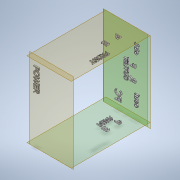
# Autodesk Inventor part: BaseTextWhite
Saved by Autodesk Inventor 2022 (Build 260153000, 153)
## iProperties
Created: 2022-01-15
Part Number: BaseTextWhite
Material: Generic
Document SubType Name: Modeling
Designer: siwat
Density: 1 g/cm^3
Appearance: Default
VLDS_Profile: Default Part
VLDS_TimeStamp: 2022-02-28
VLDS_FailCnt: 0
VLDS_AcceptCnt: 0
Author: siwat
Autodesk Inventor part; units mm, degrees
(part 1 of 2)
ref_plane "YZ Plane" through (0, 0, 0) normal (1, 0, 0) x (0, 1, 0)
ref_plane "XZ Plane" through (0, 0, 0) normal (0, 1, 0) x (-1, 0, 0)
ref_plane "XY Plane" through (0, 0, 0) normal (0, 0, 1) x (1, 0, 0)
ref_plane "Work Plane1" through (0, 0, 0) normal (0, 0, 1) x (1, 0, 0)
sketch "Sketch1" plane through (0, 0, 0) normal (0, 0, 1) x (1, 0, 0)
  line L0 (10.9128, -13.6781) -> (10.9128, -59.6425) construction
  line L1 (10.9128, -59.6425) -> (0.4914, -59.6425) construction
  line L2 (0.4914, -59.6425) -> (0.4914, -13.6781) construction
  line L3 (0.4914, -13.6781) -> (10.9128, -13.6781) construction
  spline S0 degree 2 poles (7.6875, -21.012) (7.0392, -21.012) (5.8723, -20.5501) (5.4671, -20.1368) knots 0 0 0 1 2 2 2
  spline S1 degree 2 poles (5.4671, -20.1368) (4.9565, -19.6182) (4.4298, -18.2162) (4.4298, -17.1465) knots 0 0 0 1 2 2 2
  line L4 (4.4298, -17.1465) -> (4.4298, -16.0201)
  line L5 (4.4298, -16.0201) -> (0.7021, -16.0201)
  line L6 (0.7021, -16.0201) -> (0.7021, -14.6911)
  line L7 (0.7021, -14.6911) -> (10.7021, -14.6911)
  line L8 (10.7021, -14.6911) -> (10.7021, -17.2032)
  spline S2 degree 2 poles (10.7021, -17.2032) (10.7021, -18.0947) (10.4104, -19.3426) (10.0781, -19.8207) knots 0 0 0 1 2 2 2
  spline S3 degree 2 poles (10.0781, -19.8207) (9.6972, -20.3799) (8.5222, -21.012) (7.6875, -21.012) knots 0 0 0 1 2 2 2
  spline S4 degree 2 poles (7.647, -19.6263) (8.1656, -19.6263) (8.9274, -19.2697) (9.1705, -18.905) knots 0 0 0 1 2 2 2
  spline S5 degree 2 poles (9.1705, -18.905) (9.3812, -18.589) (9.5514, -17.7462) (9.5514, -17.1222) knots 0 0 0 1 2 2 2
  line L9 (9.5514, -17.1222) -> (9.5514, -16.0201)
  line L10 (9.5514, -16.0201) -> (5.5643, -16.0201)
  line L11 (5.5643, -16.0201) -> (5.5643, -16.9277)
  spline S6 degree 2 poles (5.5643, -16.9277) (5.5643, -17.7381) (5.8236, -18.7348) (6.164, -19.059) knots 0 0 0 1 2 2 2
  spline S7 degree 2 poles (6.164, -19.059) (6.4638, -19.3588) (7.1689, -19.6263) (7.647, -19.6263) knots 0 0 0 1 2 2 2
  spline S8 degree 2 poles (9.5595, -29.3507) (8.895, -29.918) (6.9501, -30.5501) (5.7021, -30.5501) knots 0 0 0 1 2 2 2
  spline S9 degree 2 poles (5.7021, -30.5501) (4.4865, -30.5501) (2.5173, -29.9342) (1.8528, -29.3507) knots 0 0 0 1 2 2 2
  spline S10 degree 2 poles (1.8528, -29.3507) (1.1559, -28.7348) (0.4914, -27.106) (0.4914, -26.1254) knots 0 0 0 1 2 2 2
  spline S11 degree 2 poles (0.4914, -26.1254) (0.4914, -25.1125) (1.1802, -23.4917) (1.8528, -22.9002) knots 0 0 0 1 2 2 2
  spline S12 degree 2 poles (1.8528, -22.9002) (2.5173, -22.3248) (4.4703, -21.7089) (5.7021, -21.7089) knots 0 0 0 1 2 2 2
  spline S13 degree 2 poles (5.7021, -21.7089) (6.9582, -21.7089) (8.8706, -22.3329) (9.5595, -22.9083) knots 0 0 0 1 2 2 2
  spline S14 degree 2 poles (9.5595, -22.9083) (10.224, -23.4917) (10.9128, -25.1206) (10.9128, -26.1254) knots 0 0 0 1 2 2 2
  spline S15 degree 2 poles (10.9128, -26.1254) (10.9128, -27.1465) (10.1997, -28.7835) (9.5595, -29.3507) knots 0 0 0 1 2 2 2
  spline S16 degree 2 poles (5.7021, -29.1643) (6.6907, -29.1643) (8.2223, -28.7348) (8.7248, -28.3459) knots 0 0 0 1 2 2 2
  spline S17 degree 2 poles (8.7248, -28.3459) (9.2434, -27.9488) (9.7621, -26.8305) (9.7621, -26.1335) knots 0 0 0 1 2 2 2
  spline S18 degree 2 poles (9.7621, -26.1335) (9.7621, -25.4123) (9.2596, -24.3264) (8.7248, -23.9131) knots 0 0 0 1 2 2 2
  spline S19 degree 2 poles (8.7248, -23.9131) (8.2142, -23.516) (6.6745, -23.0947) (5.7021, -23.0947) knots 0 0 0 1 2 2 2
  spline S20 degree 2 poles (5.7021, -23.0947) (3.7329, -23.0947) (1.6421, -24.7478) (1.6421, -26.1335) knots 0 0 0 1 2 2 2
  spline S21 degree 2 poles (1.6421, -26.1335) (1.6421, -27.5193) (3.7329, -29.1643) (5.7021, -29.1643) knots 0 0 0 1 2 2 2
  line L12 (10.7021, -43.2162) -> (0.7021, -40.7041)
  line L13 (0.7021, -40.7041) -> (0.7021, -39.213)
  line L14 (0.7021, -39.213) -> (9.0003, -37.1789)
  line L15 (9.0003, -37.1789) -> (0.7021, -35.2016)
  line L16 (0.7021, -35.2016) -> (0.7021, -33.7267)
  line L17 (0.7021, -33.7267) -> (10.7021, -31.1741)
  line L18 (10.7021, -31.1741) -> (10.7021, -32.5436)
  line L19 (10.7021, -32.5436) -> (2.412, -34.5533)
  line L20 (2.412, -34.5533) -> (10.7021, -36.5468)
  line L21 (10.7021, -36.5468) -> (10.7021, -37.9002)
  line L22 (10.7021, -37.9002) -> (2.3147, -39.9099)
  line L23 (2.3147, -39.9099) -> (10.7021, -41.9115)
  line L24 (10.7021, -41.9115) -> (10.7021, -43.2162)
  line L25 (0.7021, -44.4075) -> (10.7021, -44.4075)
  line L26 (10.7021, -44.4075) -> (10.7021, -50.6635)
  line L27 (10.7021, -50.6635) -> (9.5189, -50.6635)
  line L28 (9.5189, -50.6635) -> (9.5189, -45.7365)
  line L29 (9.5189, -45.7365) -> (6.7799, -45.7365)
  line L30 (6.7799, -45.7365) -> (6.7799, -50.3313)
  line L31 (6.7799, -50.3313) -> (5.5967, -50.3313)
  line L32 (5.5967, -50.3313) -> (5.5967, -45.7365)
  line L33 (5.5967, -45.7365) -> (1.8852, -45.7365)
  line L34 (1.8852, -45.7365) -> (1.8852, -50.6635)
  line L35 (1.8852, -50.6635) -> (0.7021, -50.6635)
  line L36 (0.7021, -50.6635) -> (0.7021, -44.4075)
  line L37 (0.7021, -59.8613) -> (0.7021, -58.1352)
  line L38 (0.7021, -58.1352) -> (4.681, -54.9747)
  line L39 (4.681, -54.9747) -> (4.681, -53.4512)
  line L40 (4.681, -53.4512) -> (0.7021, -53.4512)
  line L41 (0.7021, -53.4512) -> (0.7021, -52.1222)
  line L42 (0.7021, -52.1222) -> (10.7021, -52.1222)
  line L43 (10.7021, -52.1222) -> (10.7021, -54.6992)
  spline S22 degree 2 poles (10.7021, -54.6992) (10.7021, -55.5582) (10.5157, -56.717) (10.1753, -57.2438) knots 0 0 0 1 2 2 2
  spline S23 degree 2 poles (10.1753, -57.2438) (9.835, -57.7705) (8.7734, -58.3783) (7.9873, -58.3783) knots 0 0 0 1 2 2 2
  spline S24 degree 2 poles (7.9873, -58.3783) (6.8933, -58.3783) (5.4104, -57.26) (5.0538, -56.3037) knots 0 0 0 1 2 2 2
  line L44 (5.0538, -56.3037) -> (0.7021, -59.8613)
  spline S25 degree 2 poles (7.882, -56.9925) (8.3196, -56.9925) (8.9922, -56.6846) (9.211, -56.3605) knots 0 0 0 1 2 2 2
  spline S26 degree 2 poles (9.211, -56.3605) (9.3974, -56.0768) (9.5514, -55.3232) (9.5514, -54.7721) knots 0 0 0 1 2 2 2
  line L45 (9.5514, -54.7721) -> (9.5514, -53.4512)
  line L46 (9.5514, -53.4512) -> (5.7912, -53.4512)
  line L47 (5.7912, -53.4512) -> (5.7912, -54.6182)
  spline S27 degree 2 poles (5.7912, -54.6182) (5.7912, -55.1935) (5.9938, -56.1092) (6.3099, -56.4253) knots 0 0 0 1 2 2 2
  spline S28 degree 2 poles (6.3099, -56.4253) (6.5854, -56.717) (7.3634, -56.9925) (7.882, -56.9925) knots 0 0 0 1 2 2 2
  point P0 (0, 0)
  constraints: 2 other
extrude "Extrusion1" add sketch "Sketch1" against normal blind 2
ref_plane "Work Plane2" through (-0.0003, -144.9621, -142.4319) normal (0, 0, -1) x (-1, 0, 0)
sketch "Sketch2" plane through (-0.0003, -144.9621, -142.4319) normal (0, 0, -1) x (-1, 0, 0)
  line L0 (-56.0033, 81.336) -> (-56.0033, 88.5078) construction
  line L1 (-56.0033, 88.5078) -> (-46.0033, 88.5078) construction
  line L2 (-46.0033, 88.5078) -> (-46.0033, 81.336) construction
  line L3 (-46.0033, 81.336) -> (-56.0033, 81.336) construction
  line L4 (-56.1337, 56.3409) -> (-56.1337, 65.1713) construction
  line L5 (-56.1337, 65.1713) -> (-45.8315, 65.1713) construction
  line L6 (-45.8315, 65.1713) -> (-45.8315, 56.3409) construction
  line L7 (-45.8315, 56.3409) -> (-56.1337, 56.3409) construction
  line L8 (-42.4083, 53.9471) -> (-42.4083, 111.4785) construction
  line L9 (-42.4083, 111.4785) -> (-33.0274, 111.4785) construction
  line L10 (-33.0274, 111.4785) -> (-33.0274, 53.9471) construction
  line L11 (-33.0274, 53.9471) -> (-42.4083, 53.9471) construction
  line L12 (-29.0759, 10.8608) -> (-29.0759, 68.3922) construction
  line L13 (-29.0759, 68.3922) -> (-19.695, 68.3922) construction
  line L14 (-19.695, 68.3922) -> (-19.695, 10.8608) construction
  line L15 (-19.695, 10.8608) -> (-29.0759, 10.8608) construction
  line L16 (-46.1337, 65.0929) -> (-46.1337, 63.3668)
  line L17 (-46.1337, 63.3668) -> (-50.1126, 60.2064)
  line L18 (-50.1126, 60.2064) -> (-50.1126, 58.6829)
  line L19 (-50.1126, 58.6829) -> (-46.1337, 58.6829)
  line L20 (-46.1337, 58.6829) -> (-46.1337, 57.3539)
  line L21 (-46.1337, 57.3539) -> (-56.1337, 57.3539)
  line L22 (-56.1337, 57.3539) -> (-56.1337, 59.9308)
  spline S0 degree 2 poles (-56.1337, 59.9308) (-56.1337, 60.7898) (-55.9473, 61.9487) (-55.6069, 62.4754) knots 0 0 0 1 2 2 2
  spline S1 degree 2 poles (-55.6069, 62.4754) (-55.2666, 63.0022) (-54.205, 63.6099) (-53.4189, 63.6099) knots 0 0 0 1 2 2 2
  spline S2 degree 2 poles (-53.4189, 63.6099) (-52.3249, 63.6099) (-50.8419, 62.4916) (-50.4854, 61.5354) knots 0 0 0 1 2 2 2
  line L23 (-50.4854, 61.5354) -> (-46.1337, 65.0929)
  spline S3 degree 2 poles (-53.3136, 62.2242) (-53.7512, 62.2242) (-54.4238, 61.9163) (-54.6426, 61.5921) knots 0 0 0 1 2 2 2
  spline S4 degree 2 poles (-54.6426, 61.5921) (-54.829, 61.3085) (-54.9829, 60.5548) (-54.9829, 60.0038) knots 0 0 0 1 2 2 2
  line L24 (-54.9829, 60.0038) -> (-54.9829, 58.6829)
  line L25 (-54.9829, 58.6829) -> (-51.2228, 58.6829)
  line L26 (-51.2228, 58.6829) -> (-51.2228, 59.8498)
  spline S5 degree 2 poles (-51.2228, 59.8498) (-51.2228, 60.4252) (-51.4254, 61.3409) (-51.7414, 61.6569) knots 0 0 0 1 2 2 2
  spline S6 degree 2 poles (-51.7414, 61.6569) (-52.017, 61.9487) (-52.7949, 62.2242) (-53.3136, 62.2242) knots 0 0 0 1 2 2 2
  line L27 (-54.8201, 88.3295) -> (-54.8201, 83.678)
  line L28 (-54.8201, 83.678) -> (-52, 83.678)
  line L29 (-52, 83.678) -> (-52, 88.135)
  line L30 (-52, 88.135) -> (-50.8169, 88.135)
  line L31 (-50.8169, 88.135) -> (-50.8169, 83.678)
  line L32 (-50.8169, 83.678) -> (-46.0033, 83.678)
  line L33 (-46.0033, 83.678) -> (-46.0033, 82.349)
  line L34 (-46.0033, 82.349) -> (-56.0033, 82.349)
  line L35 (-56.0033, 82.349) -> (-56.0033, 88.3295)
  line L36 (-56.0033, 88.3295) -> (-54.8201, 88.3295)
  spline S7 degree 2 poles (-41.3257, 60.4171) (-40.7941, 60.8709) (-39.2382, 61.3766) (-38.2398, 61.3766) knots 0 0 0 1 2 2 2
  spline S8 degree 2 poles (-38.2398, 61.3766) (-37.2673, 61.3766) (-35.692, 60.8839) (-35.1604, 60.4171) knots 0 0 0 1 2 2 2
  spline S9 degree 2 poles (-35.1604, 60.4171) (-34.6028, 59.9244) (-34.0712, 58.6213) (-34.0712, 57.8369) knots 0 0 0 1 2 2 2
  spline S10 degree 2 poles (-34.0712, 57.8369) (-34.0712, 57.0265) (-34.6223, 55.7299) (-35.1604, 55.2567) knots 0 0 0 1 2 2 2
  spline S11 degree 2 poles (-35.1604, 55.2567) (-35.692, 54.7964) (-37.2544, 54.3037) (-38.2398, 54.3037) knots 0 0 0 1 2 2 2
  spline S12 degree 2 poles (-38.2398, 54.3037) (-39.2446, 54.3037) (-40.7746, 54.8028) (-41.3257, 55.2631) knots 0 0 0 1 2 2 2
  spline S13 degree 2 poles (-41.3257, 55.2631) (-41.8573, 55.7299) (-42.4083, 57.033) (-42.4083, 57.8369) knots 0 0 0 1 2 2 2
  spline S14 degree 2 poles (-42.4083, 57.8369) (-42.4083, 58.6537) (-41.8378, 59.9633) (-41.3257, 60.4171) knots 0 0 0 1 2 2 2
  spline S15 degree 2 poles (-38.2398, 60.268) (-39.0307, 60.268) (-40.256, 59.9244) (-40.6579, 59.6132) knots 0 0 0 1 2 2 2
  spline S16 degree 2 poles (-40.6579, 59.6132) (-41.0728, 59.2956) (-41.4878, 58.4009) (-41.4878, 57.8434) knots 0 0 0 1 2 2 2
  spline S17 degree 2 poles (-41.4878, 57.8434) (-41.4878, 57.2664) (-41.0858, 56.3977) (-40.6579, 56.067) knots 0 0 0 1 2 2 2
  spline S18 degree 2 poles (-40.6579, 56.067) (-40.2495, 55.7494) (-39.0177, 55.4122) (-38.2398, 55.4122) knots 0 0 0 1 2 2 2
  spline S19 degree 2 poles (-38.2398, 55.4122) (-36.6644, 55.4122) (-34.9918, 56.7348) (-34.9918, 57.8434) knots 0 0 0 1 2 2 2
  spline S20 degree 2 poles (-34.9918, 57.8434) (-34.9918, 58.952) (-36.6644, 60.268) (-38.2398, 60.268) knots 0 0 0 1 2 2 2
  spline S21 degree 2 poles (-34.0712, 65.3377) (-34.0712, 64.631) (-34.4408, 63.5808) (-34.8103, 63.2113) knots 0 0 0 1 2 2 2
  spline S22 degree 2 poles (-34.8103, 63.2113) (-35.2252, 62.7899) (-36.3921, 62.4463) (-37.2479, 62.4463) knots 0 0 0 1 2 2 2
  line L37 (-37.2479, 62.4463) -> (-42.2398, 62.4463)
  line L38 (-42.2398, 62.4463) -> (-42.2398, 63.5095)
  line L39 (-42.2398, 63.5095) -> (-37.2479, 63.5095)
  spline S23 degree 2 poles (-37.2479, 63.5095) (-36.6904, 63.5095) (-35.9383, 63.6521) (-35.6336, 63.8531) knots 0 0 0 1 2 2 2
  spline S24 degree 2 poles (-35.6336, 63.8531) (-35.3095, 64.067) (-34.9788, 64.8061) (-34.9788, 65.3377) knots 0 0 0 1 2 2 2
  spline S25 degree 2 poles (-34.9788, 65.3377) (-34.9788, 65.8369) (-35.3095, 66.6148) (-35.6336, 66.8288) knots 0 0 0 1 2 2 2
  spline S26 degree 2 poles (-35.6336, 66.8288) (-35.9383, 67.0298) (-36.6839, 67.1724) (-37.222, 67.1724) knots 0 0 0 1 2 2 2
  line L40 (-37.222, 67.1724) -> (-42.2398, 67.1724)
  line L41 (-42.2398, 67.1724) -> (-42.2398, 68.2356)
  line L42 (-42.2398, 68.2356) -> (-37.2479, 68.2356)
  spline S27 degree 2 poles (-37.2479, 68.2356) (-36.4116, 68.2356) (-35.2187, 67.8985) (-34.8103, 67.4706) knots 0 0 0 1 2 2 2
  spline S28 degree 2 poles (-34.8103, 67.4706) (-34.4343, 67.0881) (-34.0712, 66.0768) (-34.0712, 65.3377) knots 0 0 0 1 2 2 2
  line L43 (-34.2398, 71.6262) -> (-41.2933, 71.6262)
  line L44 (-41.2933, 71.6262) -> (-41.2933, 68.9422)
  line L45 (-41.2933, 68.9422) -> (-42.2398, 68.9422)
  line L46 (-42.2398, 68.9422) -> (-42.2398, 75.3733)
  line L47 (-42.2398, 75.3733) -> (-41.2933, 75.3733)
  line L48 (-41.2933, 75.3733) -> (-41.2933, 72.6894)
  line L49 (-41.2933, 72.6894) -> (-34.2398, 72.6894)
  line L50 (-34.2398, 72.6894) -> (-34.2398, 71.6262)
  line L51 (-34.2398, 80.8191) -> (-34.2398, 76.1837)
  line L52 (-34.2398, 76.1837) -> (-42.2398, 76.1837)
  line L53 (-42.2398, 76.1837) -> (-42.2398, 77.2469)
  line L54 (-42.2398, 77.2469) -> (-35.1863, 77.2469)
  line L55 (-35.1863, 77.2469) -> (-35.1863, 80.8191)
  line L56 (-35.1863, 80.8191) -> (-34.2398, 80.8191)
  line L57 (-34.2398, 81.6554) -> (-42.2398, 81.6554)
  line L58 (-42.2398, 81.6554) -> (-42.2398, 86.6602)
  line L59 (-42.2398, 86.6602) -> (-41.2933, 86.6602)
  line L60 (-41.2933, 86.6602) -> (-41.2933, 82.7186)
  line L61 (-41.2933, 82.7186) -> (-39.102, 82.7186)
  line L62 (-39.102, 82.7186) -> (-39.102, 86.3944)
  line L63 (-39.102, 86.3944) -> (-38.1555, 86.3944)
  line L64 (-38.1555, 86.3944) -> (-38.1555, 82.7186)
  line L65 (-38.1555, 82.7186) -> (-35.1863, 82.7186)
  line L66 (-35.1863, 82.7186) -> (-35.1863, 86.6602)
  line L67 (-35.1863, 86.6602) -> (-34.2398, 86.6602)
  line L68 (-34.2398, 86.6602) -> (-34.2398, 81.6554)
  line L69 (-34.2398, 89.6943) -> (-41.2933, 89.6943)
  line L70 (-41.2933, 89.6943) -> (-41.2933, 87.0103)
  line L71 (-41.2933, 87.0103) -> (-42.2398, 87.0103)
  line L72 (-42.2398, 87.0103) -> (-42.2398, 93.4414)
  line L73 (-42.2398, 93.4414) -> (-41.2933, 93.4414)
  line L74 (-41.2933, 93.4414) -> (-41.2933, 90.7575)
  line L75 (-41.2933, 90.7575) -> (-34.2398, 90.7575)
  line L76 (-34.2398, 90.7575) -> (-34.2398, 89.6943)
  spline S29 degree 2 poles (-25.2445, 19.6615) (-24.4665, 19.6615) (-23.0662, 19.1072) (-22.58, 18.6113) knots 0 0 0 1 2 2 2
  spline S30 degree 2 poles (-22.58, 18.6113) (-21.9673, 17.9889) (-21.3352, 16.3066) (-21.3352, 15.0229) knots 0 0 0 1 2 2 2
  line L77 (-21.3352, 15.0229) -> (-21.3352, 13.6712)
  line L78 (-21.3352, 13.6712) -> (-16.862, 13.6712)
  line L79 (-16.862, 13.6712) -> (-16.862, 12.0764)
  line L80 (-16.862, 12.0764) -> (-28.862, 12.0764)
  line L81 (-28.862, 12.0764) -> (-28.862, 15.091)
  spline S31 degree 2 poles (-28.862, 15.091) (-28.862, 16.1607) (-28.5119, 17.6583) (-28.1132, 18.232) knots 0 0 0 1 2 2 2
  spline S32 degree 2 poles (-28.1132, 18.232) (-27.6561, 18.903) (-26.2461, 19.6615) (-25.2445, 19.6615) knots 0 0 0 1 2 2 2
  spline S33 degree 2 poles (-25.1959, 17.9986) (-25.8182, 17.9986) (-26.7323, 17.5707) (-27.0241, 17.1331) knots 0 0 0 1 2 2 2
  spline S34 degree 2 poles (-27.0241, 17.1331) (-27.2769, 16.7539) (-27.4811, 15.7425) (-27.4811, 14.9938) knots 0 0 0 1 2 2 2
  line L82 (-27.4811, 14.9938) -> (-27.4811, 13.6712)
  line L83 (-27.4811, 13.6712) -> (-22.6967, 13.6712)
  line L84 (-22.6967, 13.6712) -> (-22.6967, 14.7604)
  spline S35 degree 2 poles (-22.6967, 14.7604) (-22.6967, 15.7328) (-23.0079, 16.9289) (-23.4163, 17.3179) knots 0 0 0 1 2 2 2
  spline S36 degree 2 poles (-23.4163, 17.3179) (-23.7761, 17.6777) (-24.6221, 17.9986) (-25.1959, 17.9986) knots 0 0 0 1 2 2 2
  spline S37 degree 2 poles (-16.648, 25.8657) (-16.648, 24.6988) (-17.4357, 22.7247) (-18.2234, 22.0051) knots 0 0 0 1 2 2 2
  spline S38 degree 2 poles (-18.2234, 22.0051) (-19.0014, 21.2855) (-21.3352, 20.4978) (-22.8523, 20.4978) knots 0 0 0 1 2 2 2
  spline S39 degree 2 poles (-22.8523, 20.4978) (-24.3596, 20.4978) (-26.5962, 21.266) (-27.4228, 21.9954) knots 0 0 0 1 2 2 2
  spline S40 degree 2 poles (-27.4228, 21.9954) (-28.2299, 22.715) (-29.0759, 24.6793) (-29.0759, 25.8949) knots 0 0 0 1 2 2 2
  spline S41 degree 2 poles (-29.0759, 25.8949) (-29.0759, 26.4978) (-28.9009, 27.5578) (-28.7647, 28.0051) knots 0 0 0 1 2 2 2
  spline S42 degree 2 poles (-28.7647, 28.0051) (-28.6383, 28.3941) (-28.2785, 29.2012) (-28.0646, 29.5999) knots 0 0 0 1 2 2 2
  line L85 (-28.0646, 29.5999) -> (-26.1391, 29.5999)
  line L86 (-26.1391, 29.5999) -> (-26.1391, 29.4735)
  spline S43 degree 2 poles (-26.1391, 29.4735) (-26.3336, 29.2596) (-26.8782, 28.5983) (-27.1408, 28.1218) knots 0 0 0 1 2 2 2
  spline S44 degree 2 poles (-27.1408, 28.1218) (-27.3936, 27.6647) (-27.7145, 26.5853) (-27.7145, 25.8852) knots 0 0 0 1 2 2 2
  spline S45 degree 2 poles (-27.7145, 25.8852) (-27.7145, 25.1169) (-27.0824, 23.7458) (-26.4795, 23.2304) knots 0 0 0 1 2 2 2
  spline S46 degree 2 poles (-26.4795, 23.2304) (-25.8668, 22.7247) (-24.0095, 22.1607) (-22.8523, 22.1607) knots 0 0 0 1 2 2 2
  spline S47 degree 2 poles (-22.8523, 22.1607) (-21.6173, 22.1607) (-19.8377, 22.7539) (-19.225, 23.2693) knots 0 0 0 1 2 2 2
  spline S48 degree 2 poles (-19.225, 23.2693) (-18.6318, 23.775) (-18.0289, 25.1267) (-18.0289, 25.8852) knots 0 0 0 1 2 2 2
  spline S49 degree 2 poles (-18.0289, 25.8852) (-18.0289, 26.5756) (-18.3693, 27.7523) (-18.6221, 28.2093) knots 0 0 0 1 2 2 2
  spline S50 degree 2 poles (-18.6221, 28.2093) (-18.8749, 28.6469) (-19.4001, 29.2985) (-19.5848, 29.4832) knots 0 0 0 1 2 2 2
  line L87 (-19.5848, 29.4832) -> (-19.5848, 29.5999)
  line L88 (-19.5848, 29.5999) -> (-17.6788, 29.5999)
  spline S51 degree 2 poles (-17.6788, 29.5999) (-17.4941, 29.2012) (-17.1537, 28.501) (-16.9981, 28.0051) knots 0 0 0 1 2 2 2
  spline S52 degree 2 poles (-16.9981, 28.0051) (-16.8231, 27.48) (-16.648, 26.5853) (-16.648, 25.8657) knots 0 0 0 1 2 2 2
  point P0 (-0.0003, 144.9621)
  constraints: 8 other
extrude "Extrusion2" add sketch "Sketch2" against normal blind 2
ref_plane "Work Plane3" through (-0.0003, -144.9621, 0) normal (0, -1, 0) x (-0.0016, 0, -1)
sketch "Sketch3" plane through (-0.0003, -144.9621, 0) normal (0, -1, 0) x (-0.0016, 0, -1)
  line L0 (112.8578, 52.4306) -> (120.805, 52.4306) construction
  line L1 (120.805, 52.4306) -> (120.805, 40.8515) construction
  line L2 (120.805, 40.8515) -> (112.8578, 40.8515) construction
  line L3 (112.8578, 40.8515) -> (112.8578, 52.4306) construction
  line L4 (88.4254, 52.4306) -> (96.3726, 52.4306) construction
  line L5 (96.3726, 52.4306) -> (96.3726, 40.8515) construction
  line L6 (96.3726, 40.8515) -> (88.4254, 40.8515) construction
  line L7 (88.4254, 40.8515) -> (88.4254, 52.4306) construction
  line L8 (91.0018, 27.1747) -> (91.0018, 38.3124) construction
  line L9 (91.0018, 38.3124) -> (117.8911, 38.3124) construction
  line L10 (117.8911, 38.3124) -> (117.8911, 27.1747) construction
  line L11 (117.8911, 27.1747) -> (91.0018, 27.1747) construction
  line L12 (89.4383, 42.4306) -> (89.4383, 52.4306)
  line L13 (89.4383, 52.4306) -> (95.6944, 52.4306)
  line L14 (95.6944, 52.4306) -> (95.6944, 51.2474)
  line L15 (95.6944, 51.2474) -> (90.7673, 51.2474)
  line L16 (90.7673, 51.2474) -> (90.7673, 48.5084)
  line L17 (90.7673, 48.5084) -> (95.3622, 48.5084)
  line L18 (95.3622, 48.5084) -> (95.3622, 47.3252)
  line L19 (95.3622, 47.3252) -> (90.7673, 47.3252)
  line L20 (90.7673, 47.3252) -> (90.7673, 43.6137)
  line L21 (90.7673, 43.6137) -> (95.6944, 43.6137)
  line L22 (95.6944, 43.6137) -> (95.6944, 42.4306)
  line L23 (95.6944, 42.4306) -> (89.4383, 42.4306)
  spline S0 degree 2 poles (120.1917, 49.416) (120.1917, 48.7677) (119.7298, 47.6008) (119.3165, 47.1956) knots 0 0 0 1 2 2 2
  spline S1 degree 2 poles (119.3165, 47.1956) (118.7978, 46.685) (117.3959, 46.1583) (116.3262, 46.1583) knots 0 0 0 1 2 2 2
  line L24 (116.3262, 46.1583) -> (115.1998, 46.1583)
  line L25 (115.1998, 46.1583) -> (115.1998, 42.4306)
  line L26 (115.1998, 42.4306) -> (113.8708, 42.4306)
  line L27 (113.8708, 42.4306) -> (113.8708, 52.4306)
  line L28 (113.8708, 52.4306) -> (116.3829, 52.4306)
  spline S2 degree 2 poles (116.3829, 52.4306) (117.2743, 52.4306) (118.5223, 52.1388) (119.0004, 51.8066) knots 0 0 0 1 2 2 2
  spline S3 degree 2 poles (119.0004, 51.8066) (119.5596, 51.4257) (120.1917, 50.2507) (120.1917, 49.416) knots 0 0 0 1 2 2 2
  spline S4 degree 2 poles (118.8059, 49.3755) (118.8059, 49.8941) (118.4494, 50.6559) (118.0847, 50.899) knots 0 0 0 1 2 2 2
  spline S5 degree 2 poles (118.0847, 50.899) (117.7687, 51.1097) (116.9259, 51.2799) (116.3019, 51.2799) knots 0 0 0 1 2 2 2
  line L29 (116.3019, 51.2799) -> (115.1998, 51.2799)
  line L30 (115.1998, 51.2799) -> (115.1998, 47.2928)
  line L31 (115.1998, 47.2928) -> (116.1074, 47.2928)
  spline S6 degree 2 poles (116.1074, 47.2928) (116.9178, 47.2928) (117.9145, 47.5521) (118.2387, 47.8925) knots 0 0 0 1 2 2 2
  spline S7 degree 2 poles (118.2387, 47.8925) (118.5385, 48.1923) (118.8059, 48.8974) (118.8059, 49.3755) knots 0 0 0 1 2 2 2
  line L32 (98.468, 30.3124) -> (97.0872, 30.3124)
  line L33 (97.0872, 30.3124) -> (94.5588, 33.4955)
  line L34 (94.5588, 33.4955) -> (93.34, 33.4955)
  line L35 (93.34, 33.4955) -> (93.34, 30.3124)
  line L36 (93.34, 30.3124) -> (92.2768, 30.3124)
  line L37 (92.2768, 30.3124) -> (92.2768, 38.3124)
  line L38 (92.2768, 38.3124) -> (94.3384, 38.3124)
  spline S8 degree 2 poles (94.3384, 38.3124) (95.0256, 38.3124) (95.9526, 38.1633) (96.374, 37.891) knots 0 0 0 1 2 2 2
  spline S9 degree 2 poles (96.374, 37.891) (96.7954, 37.6187) (97.2817, 36.7694) (97.2817, 36.1406) knots 0 0 0 1 2 2 2
  spline S10 degree 2 poles (97.2817, 36.1406) (97.2817, 35.2654) (96.387, 34.079) (95.622, 33.7937) knots 0 0 0 1 2 2 2
  line L39 (95.622, 33.7937) -> (98.468, 30.3124)
  spline S11 degree 2 poles (96.1731, 36.0563) (96.1731, 36.4064) (95.9267, 36.9445) (95.6674, 37.1195) knots 0 0 0 1 2 2 2
  spline S12 degree 2 poles (95.6674, 37.1195) (95.4405, 37.2686) (94.8376, 37.3918) (94.3967, 37.3918) knots 0 0 0 1 2 2 2
  line L40 (94.3967, 37.3918) -> (93.34, 37.3918)
  line L41 (93.34, 37.3918) -> (93.34, 34.3837)
  line L42 (93.34, 34.3837) -> (94.2735, 34.3837)
  spline S13 degree 2 poles (94.2735, 34.3837) (94.7338, 34.3837) (95.4664, 34.5457) (95.7193, 34.7986) knots 0 0 0 1 2 2 2
  spline S14 degree 2 poles (95.7193, 34.7986) (95.9526, 35.019) (96.1731, 35.6414) (96.1731, 36.0563) knots 0 0 0 1 2 2 2
  line L43 (99.1034, 30.3124) -> (99.1034, 38.3124)
  line L44 (99.1034, 38.3124) -> (104.1082, 38.3124)
  line L45 (104.1082, 38.3124) -> (104.1082, 37.3658)
  line L46 (104.1082, 37.3658) -> (100.1666, 37.3658)
  line L47 (100.1666, 37.3658) -> (100.1666, 35.1746)
  line L48 (100.1666, 35.1746) -> (103.8424, 35.1746)
  line L49 (103.8424, 35.1746) -> (103.8424, 34.2281)
  line L50 (103.8424, 34.2281) -> (100.1666, 34.2281)
  line L51 (100.1666, 34.2281) -> (100.1666, 31.2589)
  line L52 (100.1666, 31.2589) -> (104.1082, 31.2589)
  line L53 (104.1082, 31.2589) -> (104.1082, 30.3124)
  line L54 (104.1082, 30.3124) -> (99.1034, 30.3124)
  line L55 (104.4129, 30.3124) -> (107.1099, 38.3124)
  line L56 (107.1099, 38.3124) -> (108.4194, 38.3124)
  line L57 (108.4194, 38.3124) -> (111.1163, 30.3124)
  line L58 (111.1163, 30.3124) -> (109.9948, 30.3124)
  line L59 (109.9948, 30.3124) -> (109.2687, 32.549)
  line L60 (109.2687, 32.549) -> (106.2152, 32.549)
  line L61 (106.2152, 32.549) -> (105.4891, 30.3124)
  line L62 (105.4891, 30.3124) -> (104.4129, 30.3124)
  line L63 (108.977, 33.4566) -> (107.7387, 37.2232)
  line L64 (107.7387, 37.2232) -> (106.5069, 33.4566)
  line L65 (106.5069, 33.4566) -> (108.977, 33.4566)
  line L66 (118.0661, 30.3124) -> (116.6852, 30.3124)
  line L67 (116.6852, 30.3124) -> (114.1569, 33.4955)
  line L68 (114.1569, 33.4955) -> (112.9381, 33.4955)
  line L69 (112.9381, 33.4955) -> (112.9381, 30.3124)
  line L70 (112.9381, 30.3124) -> (111.8748, 30.3124)
  line L71 (111.8748, 30.3124) -> (111.8748, 38.3124)
  line L72 (111.8748, 38.3124) -> (113.9364, 38.3124)
  spline S15 degree 2 poles (113.9364, 38.3124) (114.6236, 38.3124) (115.5507, 38.1633) (115.9721, 37.891) knots 0 0 0 1 2 2 2
  spline S16 degree 2 poles (115.9721, 37.891) (116.3935, 37.6187) (116.8797, 36.7694) (116.8797, 36.1406) knots 0 0 0 1 2 2 2
  spline S17 degree 2 poles (116.8797, 36.1406) (116.8797, 35.2654) (115.9851, 34.079) (115.2201, 33.7937) knots 0 0 0 1 2 2 2
  line L73 (115.2201, 33.7937) -> (118.0661, 30.3124)
  spline S18 degree 2 poles (115.7711, 36.0563) (115.7711, 36.4064) (115.5248, 36.9445) (115.2654, 37.1195) knots 0 0 0 1 2 2 2
  spline S19 degree 2 poles (115.2654, 37.1195) (115.0385, 37.2686) (114.4356, 37.3918) (113.9948, 37.3918) knots 0 0 0 1 2 2 2
  line L74 (113.9948, 37.3918) -> (112.9381, 37.3918)
  line L75 (112.9381, 37.3918) -> (112.9381, 34.3837)
  line L76 (112.9381, 34.3837) -> (113.8716, 34.3837)
  spline S20 degree 2 poles (113.8716, 34.3837) (114.3319, 34.3837) (115.0645, 34.5457) (115.3173, 34.7986) knots 0 0 0 1 2 2 2
  spline S21 degree 2 poles (115.3173, 34.7986) (115.5507, 35.019) (115.7711, 35.6414) (115.7711, 36.0563) knots 0 0 0 1 2 2 2
  point P0 (0, 0)
  constraints: 2 collinear, 6 other
extrude "Extrusion3" add sketch "Sketch3" against normal blind 2
ref_plane "Work Plane4" through (0, 0, -142.4319) normal (0, 1, 0) x (0.0016, 0, 1)
sketch "Sketch4" plane through (0, 0, -142.4319) normal (0, 1, 0) x (0.0016, 0, 1)
  line L0 (23.3168, 51.6972) -> (31.264, 51.6972) construction
  line L1 (31.264, 51.6972) -> (31.264, 36.0773) construction
  line L2 (31.264, 36.0773) -> (23.3168, 36.0773) construction
  line L3 (23.3168, 36.0773) -> (23.3168, 51.6972) construction
  line L4 (46.1036, 51.6972) -> (54.0508, 51.6972) construction
  line L5 (54.0508, 51.6972) -> (54.0508, 36.0773) construction
  line L6 (54.0508, 36.0773) -> (46.1036, 36.0773) construction
  line L7 (46.1036, 36.0773) -> (46.1036, 51.6972) construction
  line L8 (63.0369, 69.0082) -> (98.918, 69.0082) construction
  line L9 (98.918, 69.0082) -> (98.918, 60.9691) construction
  line L10 (98.918, 60.9691) -> (63.0369, 60.9691) construction
  line L11 (63.0369, 60.9691) -> (63.0369, 69.0082) construction
  line L12 (47.1166, 41.6972) -> (47.1166, 51.6972)
  line L13 (47.1166, 51.6972) -> (53.3727, 51.6972)
  line L14 (53.3727, 51.6972) -> (53.3727, 50.514)
  line L15 (53.3727, 50.514) -> (48.4456, 50.514)
  line L16 (48.4456, 50.514) -> (48.4456, 47.775)
  line L17 (48.4456, 47.775) -> (53.0404, 47.775)
  line L18 (53.0404, 47.775) -> (53.0404, 46.5918)
  line L19 (53.0404, 46.5918) -> (48.4456, 46.5918)
  line L20 (48.4456, 46.5918) -> (48.4456, 42.8803)
  line L21 (48.4456, 42.8803) -> (53.3727, 42.8803)
  line L22 (53.3727, 42.8803) -> (53.3727, 41.6972)
  line L23 (53.3727, 41.6972) -> (47.1166, 41.6972)
  spline S0 degree 2 poles (30.6507, 48.6826) (30.6507, 48.0343) (30.1887, 46.8674) (29.7754, 46.4622) knots 0 0 0 1 2 2 2
  spline S1 degree 2 poles (29.7754, 46.4622) (29.2568, 45.9516) (27.8549, 45.4249) (26.7852, 45.4249) knots 0 0 0 1 2 2 2
  line L24 (26.7852, 45.4249) -> (25.6588, 45.4249)
  line L25 (25.6588, 45.4249) -> (25.6588, 41.6972)
  line L26 (25.6588, 41.6972) -> (24.3297, 41.6972)
  line L27 (24.3297, 41.6972) -> (24.3297, 51.6972)
  line L28 (24.3297, 51.6972) -> (26.8419, 51.6972)
  spline S2 degree 2 poles (26.8419, 51.6972) (27.7333, 51.6972) (28.9813, 51.4055) (29.4594, 51.0732) knots 0 0 0 1 2 2 2
  spline S3 degree 2 poles (29.4594, 51.0732) (30.0186, 50.6923) (30.6507, 49.5173) (30.6507, 48.6826) knots 0 0 0 1 2 2 2
  spline S4 degree 2 poles (29.2649, 48.6421) (29.2649, 49.1607) (28.9084, 49.9225) (28.5437, 50.1656) knots 0 0 0 1 2 2 2
  spline S5 degree 2 poles (28.5437, 50.1656) (28.2276, 50.3763) (27.3848, 50.5465) (26.7609, 50.5465) knots 0 0 0 1 2 2 2
  line L29 (26.7609, 50.5465) -> (25.6588, 50.5465)
  line L30 (25.6588, 50.5465) -> (25.6588, 46.5594)
  line L31 (25.6588, 46.5594) -> (26.5664, 46.5594)
  spline S6 degree 2 poles (26.5664, 46.5594) (27.3767, 46.5594) (28.3735, 46.8187) (28.6977, 47.1591) knots 0 0 0 1 2 2 2
  spline S7 degree 2 poles (28.6977, 47.1591) (28.9975, 47.4589) (29.2649, 48.164) (29.2649, 48.6421) knots 0 0 0 1 2 2 2
  line L32 (68.6317, 67.8932) -> (64.9105, 67.8932)
  line L33 (64.9105, 67.8932) -> (64.9105, 65.6371)
  line L34 (64.9105, 65.6371) -> (68.4761, 65.6371)
  line L35 (68.4761, 65.6371) -> (68.4761, 64.6906)
  line L36 (68.4761, 64.6906) -> (64.9105, 64.6906)
  line L37 (64.9105, 64.6906) -> (64.9105, 60.8397)
  line L38 (64.9105, 60.8397) -> (63.8473, 60.8397)
  line L39 (63.8473, 60.8397) -> (63.8473, 68.8397)
  line L40 (63.8473, 68.8397) -> (68.6317, 68.8397)
  line L41 (68.6317, 68.8397) -> (68.6317, 67.8932)
  line L42 (75.7759, 60.8397) -> (74.3951, 60.8397)
  line L43 (74.3951, 60.8397) -> (71.8667, 64.0228)
  line L44 (71.8667, 64.0228) -> (70.6479, 64.0228)
  line L45 (70.6479, 64.0228) -> (70.6479, 60.8397)
  line L46 (70.6479, 60.8397) -> (69.5847, 60.8397)
  line L47 (69.5847, 60.8397) -> (69.5847, 68.8397)
  line L48 (69.5847, 68.8397) -> (71.6463, 68.8397)
  spline S8 degree 2 poles (71.6463, 68.8397) (72.3335, 68.8397) (73.2606, 68.6906) (73.6819, 68.4183) knots 0 0 0 1 2 2 2
  spline S9 degree 2 poles (73.6819, 68.4183) (74.1033, 68.146) (74.5896, 67.2967) (74.5896, 66.6679) knots 0 0 0 1 2 2 2
  spline S10 degree 2 poles (74.5896, 66.6679) (74.5896, 65.7927) (73.6949, 64.6063) (72.9299, 64.3211) knots 0 0 0 1 2 2 2
  line L49 (72.9299, 64.3211) -> (75.7759, 60.8397)
  spline S11 degree 2 poles (73.481, 66.5836) (73.481, 66.9337) (73.2346, 67.4718) (72.9753, 67.6468) knots 0 0 0 1 2 2 2
  spline S12 degree 2 poles (72.9753, 67.6468) (72.7484, 67.7959) (72.1455, 67.9191) (71.7046, 67.9191) knots 0 0 0 1 2 2 2
  line L50 (71.7046, 67.9191) -> (70.6479, 67.9191)
  line L51 (70.6479, 67.9191) -> (70.6479, 64.911)
  line L52 (70.6479, 64.911) -> (71.5815, 64.911)
  spline S13 degree 2 poles (71.5815, 64.911) (72.0418, 64.911) (72.7743, 65.0731) (73.0272, 65.3259) knots 0 0 0 1 2 2 2
  spline S14 degree 2 poles (73.0272, 65.3259) (73.2606, 65.5463) (73.481, 66.1687) (73.481, 66.5836) knots 0 0 0 1 2 2 2
  spline S15 degree 2 poles (82.0709, 67.9256) (82.5247, 67.394) (83.0304, 65.8381) (83.0304, 64.8397) knots 0 0 0 1 2 2 2
  spline S16 degree 2 poles (83.0304, 64.8397) (83.0304, 63.8672) (82.5377, 62.2919) (82.0709, 61.7603) knots 0 0 0 1 2 2 2
  spline S17 degree 2 poles (82.0709, 61.7603) (81.5782, 61.2027) (80.2751, 60.6711) (79.4907, 60.6711) knots 0 0 0 1 2 2 2
  spline S18 degree 2 poles (79.4907, 60.6711) (78.6803, 60.6711) (77.3837, 61.2222) (76.9105, 61.7603) knots 0 0 0 1 2 2 2
  spline S19 degree 2 poles (76.9105, 61.7603) (76.4502, 62.2919) (75.9575, 63.8543) (75.9575, 64.8397) knots 0 0 0 1 2 2 2
  spline S20 degree 2 poles (75.9575, 64.8397) (75.9575, 65.8446) (76.4567, 67.3745) (76.917, 67.9256) knots 0 0 0 1 2 2 2
  spline S21 degree 2 poles (76.917, 67.9256) (77.3837, 68.4572) (78.6868, 69.0082) (79.4907, 69.0082) knots 0 0 0 1 2 2 2
  spline S22 degree 2 poles (79.4907, 69.0082) (80.3076, 69.0082) (81.6171, 68.4377) (82.0709, 67.9256) knots 0 0 0 1 2 2 2
  spline S23 degree 2 poles (81.9218, 64.8397) (81.9218, 65.6306) (81.5782, 66.8559) (81.267, 67.2578) knots 0 0 0 1 2 2 2
  spline S24 degree 2 poles (81.267, 67.2578) (80.9494, 67.6728) (80.0547, 68.0877) (79.4972, 68.0877) knots 0 0 0 1 2 2 2
  spline S25 degree 2 poles (79.4972, 68.0877) (78.9202, 68.0877) (78.0515, 67.6857) (77.7208, 67.2578) knots 0 0 0 1 2 2 2
  spline S26 degree 2 poles (77.7208, 67.2578) (77.4032, 66.8494) (77.0661, 65.6176) (77.0661, 64.8397) knots 0 0 0 1 2 2 2
  spline S27 degree 2 poles (77.0661, 64.8397) (77.0661, 63.2643) (78.3886, 61.5917) (79.4972, 61.5917) knots 0 0 0 1 2 2 2
  spline S28 degree 2 poles (79.4972, 61.5917) (80.6058, 61.5917) (81.9218, 63.2643) (81.9218, 64.8397) knots 0 0 0 1 2 2 2
  line L53 (89.9218, 60.8397) -> (88.7289, 60.8397)
  line L54 (88.7289, 60.8397) -> (85.1892, 67.7376)
  line L55 (85.1892, 67.7376) -> (85.1892, 60.8397)
  line L56 (85.1892, 60.8397) -> (84.1973, 60.8397)
  line L57 (84.1973, 60.8397) -> (84.1973, 68.8397)
  line L58 (84.1973, 68.8397) -> (85.7079, 68.8397)
  line L59 (85.7079, 68.8397) -> (88.9299, 62.5058)
  line L60 (88.9299, 62.5058) -> (88.9299, 68.8397)
  line L61 (88.9299, 68.8397) -> (89.9218, 68.8397)
  line L62 (89.9218, 68.8397) -> (89.9218, 60.8397)
  line L63 (93.4097, 60.8397) -> (93.4097, 67.8932)
  line L64 (93.4097, 67.8932) -> (90.7257, 67.8932)
  line L65 (90.7257, 67.8932) -> (90.7257, 68.8397)
  line L66 (90.7257, 68.8397) -> (97.1568, 68.8397)
  line L67 (97.1568, 68.8397) -> (97.1568, 67.8932)
  line L68 (97.1568, 67.8932) -> (94.4729, 67.8932)
  line L69 (94.4729, 67.8932) -> (94.4729, 60.8397)
  line L70 (94.4729, 60.8397) -> (93.4097, 60.8397)
  point P0 (142.4317, -0.2259)
  constraints: 2 collinear, 6 other
extrude "Extrusion4" add sketch "Sketch4" against normal blind 2
ref_plane "Work Plane5" through (-0.0003, -144.9621, -142.4319) normal (0, 0, -1) x (-1, 0, 0)